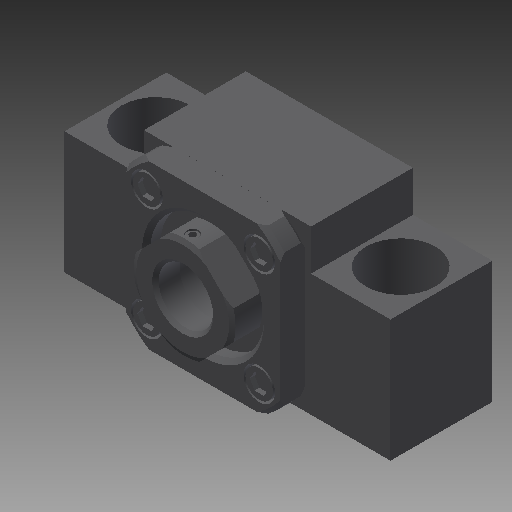
# Autodesk Inventor part: BK 15
Saved by Autodesk Inventor 2018 (Build 220112000, 112)
## iProperties
Category: PARTsolutions
Company: THK
Created: 2017-05-30
Part Number: BK 15
Catalog Web Link: www.cadenas.de
Description: Fixed Side type BK-
Vendor: THK
Document SubType Name: Modeling
Designer: psAdmin
Manufacturer: THK
Mass: 63.686 g
Surface Area: 225.318 cm^2
Volume: 63.686 cm^3
Density: 1 g/cm^3
Material: Generic
Appearance: PSOLRGB-192-192-192
PSOL_IDENT_0: {$CADENAS_DATA\23d-libs\thk\fed_screw\ball_screw\ball_screw_peripheral\suport_unit\fixed_side_type_b
PSOL_IDENT_1: k.prj},164 {VTYP=3D},{NB=BK 15},{LINA=BK 15},{NN=Fixed Side type BK},{DATE=16.05.2017 06:09:49},{GEO
PSOL_IDENT_2: MDATE=23.05.2016 07:00:00},{VERSION=},{LINEID=30},{LINESUBID=-1},{WBVAR=}  {NB=BK 15},{LINA=BK 15},{
PSOL_IDENT_3: KT=DUMMY},{IDNR=},{MN=BK 15},{SD=15.000},{L=27.000},{L1=6.000},{L2=32.000},{L3=6.000},{B=70.000},{H=
PSOL_IDENT_4: 48.000},{SB=35.000},{SH1=28.000},{B1=40.000},{H1=38.000},{E=18.000},{P=54.000},{C1=15.000},{C2=6.000
PSOL_IDENT_5: },{SD3=5.500},{SD1=6.600},{SD2=11.000},{SH=6.500},{NDM=3.000},{T=22.000},{DK=30.000},{L4=3.500},{SD4=
PSOL_IDENT_6: 19.500},{D=28.000},{DD=25.000},{P1=1.500},{PCD=39.000},{PCD1=49.500},{B2=38.000},{D1=7.800},{WF=4.00
PSOL_IDENT_7: 0},{WF1=1.500},{R3=25.000}
NN: Fixed side type BK
NB: BK 15
NBSYN: $MN.
LINA: BK 15
MN: BK 15
SUPPLIER: THK
ARTICLENO: BK 15
BOMINFO: BK 15
CREATOR: CADENAS GmbH
Title: BK 15
Author: Cadenas PARTsolutions
Autodesk Inventor part; units mm, degrees
sketch "Sketch_1" plane through (0, 0, 0) normal (0, 0, 1) x (1, 0, 0)
  line L0 (-40, -20) -> (40, -20)
  line L1 (40, -20) -> (40, 10)
  line L2 (40, 10) -> (20.5, 10)
  line L3 (20.5, 10) -> (20.5, 20)
  line L4 (20.5, 20) -> (-20.5, 20)
  line L5 (-20.5, 20) -> (-20.5, 10)
  line L6 (-20.5, 10) -> (-40, 10)
  line L7 (-40, 10) -> (-40, -20)
  line L8 (0, 20) -> (0, -20) construction
  line L9 (0, 20) -> (0, 0) construction
  dimension "d87" = 80
  dimension "d88" = 40
  dimension "d90" = 41
  dimension "d98" = 20
  dimension "d108" = 10
  constraints: 20 end point, 4 vertical, 2 horizontal, 2 midpoint, 1 collinear, 1 perpendicular, 1 other
  measures "d87" distance between parallel lines of L7 L1
  measures "d88" distance between parallel lines of L0 L4
  measures "d90" distance of L3.end L4.end
  measures "d98" distance from line of L9.end L4
  measures "d108" distance between parallel lines of L4 L2
extrude "Extrusion1" add sketch "Sketch_1" against normal blind 25
sketch "Sketch2" plane through (20.5, 10, 0) normal (0, 1, 0) x (1, 0, 0)
  line L0 (9.5, 12.5) -> (19.5, 12.5) construction
  line L1 (19.5, 0) -> (19.5, 25) projected
  dimension "d97" = 10
  constraints: 2 end point, 1 horizontal, 1 midpoint
  measures "d97" distance of L0.start L0.end
hole "Hole1" at (30, 10, -12.5) direction (0, -1, 0) diameter 11 end through all counterbore diameter 17 counterbore depth 15
sketch "Sketch_10" plane through (0, 0, 0) normal (0, 0, 1) x (1, 0, 0)
  line L0 (-19, 20) -> (-19, -20)
  line L1 (-19, -20) -> (19, -20)
  line L2 (19, -20) -> (19, 20)
  line L3 (19, 20) -> (-19, 20)
  constraints: 8 end point
extrude "Extrusion2" add sketch "Sketch_10" along normal blind 2.5
sketch "Sketch_13" plane through (0, 0, 0) normal (1, 0, 0) x (0, 1, 0)
  line L0 (0, 2.5) -> (0, 11)
  line L1 (0, 11) -> (12.5, 11)
  line L2 (12.5, 11) -> (12.5, 3.5)
  line L3 (12.5, 3.5) -> (10, 3.5)
  line L4 (10, 3.5) -> (10, 3)
  line L5 (10, 3) -> (9, 3)
  line L6 (9, 3) -> (9, 2.5)
  line L7 (9, 2.5) -> (0, 2.5)
  line L8 (0, 2.5) -> (0, 11)
  constraints: 18 end point
revolve "Revolution1" add sketch "Sketch_13" angle 360 about axis through (0, 0, 2.5) along (0, 0, -1)
sketch "Sketch_11" plane through (0, 0, 11) normal (0, 0, 1) x (1, 0, 0)
  line L0 (-22, 22) -> (-22, -22)
  line L1 (-22, -22) -> (22, -22)
  line L2 (22, -22) -> (22, 22)
  line L3 (22, 22) -> (-22, 22)
  line L4 (-15.5563, 0) -> (0, -15.5563)
  line L5 (0, -15.5563) -> (15.5563, 0)
  line L6 (15.5563, 0) -> (0, 15.5563)
  line L7 (0, 15.5563) -> (-15.5563, 0)
  constraints: 16 end point
extrude "Extrusion3" cut sketch "Sketch_11" against normal blind 8.5
sketch "Sketch_12" plane through (0, 0, 2.5) normal (0, 0, 1) x (1, 0, 0)
  line L0 (-19, 20) -> (-19, -20)
  line L1 (-19, -20) -> (19, -20)
  line L2 (19, -20) -> (19, 20)
  line L3 (19, 20) -> (-19, 20)
  circle A0 centre (0, 0) radius 14
  line L4 (-19, 20) -> (19, 20) projected
  line L5 (0, 20) -> (0, 20) construction
  line L6 (-20.5, 20) -> (20.5, 20) projected
  dimension "d91" = 28
  dimension "d92" = 38
  dimension "d93" = 38
  dimension "d94" = 40
  dimension "d95" = 40
  constraints: 10 end point, 2 midpoint, 1 centre point, 1 vertical
  measures "d91" diameter of A0
  measures "d92" distance of L2.end L0.start
  measures "d93" distance of L0.end L1.end
  measures "d94" distance of L0.start L0.end
  measures "d95" distance of L1.end L2.end
extrude "Extrusion4" add sketch "Sketch_12" along normal blind 3.5
sketch "Sketch_14" plane through (0, 0, 0) normal (1, 0, 0) x (0, 1, 0)
  line L0 (0, -50) -> (0, 50)
  line L1 (15, 6) -> (14, 6)
  line L2 (14, 6) -> (14, 5)
  line L3 (14, 5) -> (15, 6)
  constraints: 8 end point
revolve "Revolution2" cut sketch "Sketch_14" angle 360 about axis through (0, 0, -50) along (0, 0, -1)
sketch "Sketch11" plane through (0, 0, -25) normal (0, 0, -1) x (-1, 0, 0)
  point P0 (0, 0)
hole "Hole5" at (0, 0, -25) direction (0, 0, 1) diameter 15 depth 30 counterbore diameter 19.5 counterbore depth 6
sketch "Sketch_16" plane through (0, 0, 0) normal (1, 0, 0) x (0, 1, 0)
  line L0 (0, 2.5) -> (0, 11)
  line L1 (0, 11) -> (7.5, 11)
  line L2 (7.5, 11) -> (6.688, 10.188)
  line L3 (6.688, 10.188) -> (6.688, 3.312)
  line L4 (6.688, 3.312) -> (7.5, 2.5)
  line L5 (7.5, 2.5) -> (0, 2.5)
  line L6 (0, 2.5) -> (0, 11)
  constraints: 14 end point
revolve "Revolution3" cut sketch "Sketch_16" angle 360 about axis through (0, 0, 2.5) along (0, 0, -1)
thread "Thread1" size "M15x1.5" class "6H" standard "ISO Metric profile" full length
sketch "Sketch_17" plane through (0, 0, 0) normal (1, 0, 0) x (0, 1, 0)
  line L0 (0, -50) -> (0, 50)
  line L1 (14.05, 0) -> (14, 0)
  line L2 (14, 0) -> (14, -27)
  line L3 (14, -27) -> (14.05, -27)
  line L4 (14.05, -27) -> (14.05, 0)
  constraints: 10 end point
revolve "Revolution4" cut sketch "Sketch_17" angle 360 about axis through (0, 0, -50) along (0, 0, -1)
sketch "Sketch_18" plane through (0, 0, 0) normal (0.7071068, -0.7071068, 0) x (0, 0, -1)
  line L0 (-3, 19.5) -> (-6, 19.5)
  line L1 (-6, 19.5) -> (-6, 23.4)
  line L2 (-6, 23.4) -> (-3, 23.4)
  line L3 (-3, 23.4) -> (-3, 19.5)
  line L4 (-3, 19.5) -> (-6, 19.5)
  constraints: 10 end point
revolve "Revolution5" cut sketch "Sketch_18" angle 360 about axis through (13.7886, 13.7886, 3) along (0, 0, -1)
pattern_linear "Rectangular Pattern1" count 2 spacing 27.5772 along (-1, 0, 0) count 2 spacing 27.5772 along (0, -1, 0) of "Revolution5"
sketch "Sketch_20" plane through (0, 0, 0) normal (0.7071068, -0.7071068, 0) x (0, 0, -1)
  line L0 (-3, 19.5) -> (-6, 19.5)
  line L1 (-6, 19.5) -> (-6, 22.9)
  line L2 (-6, 22.9) -> (-3, 22.9)
  line L3 (-3, 22.9) -> (-3, 19.5)
  line L4 (-3, 19.5) -> (-6, 19.5)
  constraints: 10 end point
revolve "Revolution6" add sketch "Sketch_20" angle 360 about axis through (13.7886, 13.7886, 3) along (0, 0, -1)
pattern_linear "Rectangular Pattern2" count 2 spacing 27.5772 along (-1, 0, 0) count 2 spacing 27.5772 along (0, -1, 0) of "Revolution6"
sketch "Sketch_22" plane through (0, 0, 6) normal (0, 0, 1) x (0.7071068, 0.7071068, 0)
  line L0 (17.2693, -0.5977) -> (18.9023, -2.2307)
  line L1 (18.9023, -2.2307) -> (21.133, -1.633)
  line L2 (21.133, -1.633) -> (21.7307, 0.5977)
  line L3 (21.7307, 0.5977) -> (20.0977, 2.2307)
  line L4 (20.0977, 2.2307) -> (17.867, 1.633)
  line L5 (17.867, 1.633) -> (17.2693, -0.5977)
  constraints: 12 end point
extrude "Extrusion5" cut sketch "Sketch_22" against normal blind 1.2
pattern_linear "Rectangular Pattern3" count 2 spacing 27.5772 along (-1, 0, 0) count 2 spacing 27.5772 along (0, -1, 0) of "Extrusion5"
sketch "Sketch_24" plane through (0, 0, 0) normal (1, 0, 0) x (0, 1, 0)
  line L0 (12.5, 8.5) -> (7.5, 8.5)
  line L1 (7.5, 8.5) -> (7.5, 10)
  line L2 (7.5, 10) -> (12.5, 10)
  line L3 (12.5, 10) -> (12.5, 8.5)
  line L4 (12.5, 8.5) -> (7.5, 8.5)
  constraints: 10 end point
revolve "Revolution7" cut sketch "Sketch_24" angle 360 about axis through (0, 12.5, 8.5) along (0, 1, 0)
sketch "Sketch_25" plane through (0, 0, 0) normal (1, 0, 0) x (0, 1, 0)
  line L0 (12.3, 8.5) -> (8.8, 8.5)
  line L1 (8.8, 8.5) -> (8.8, 10)
  line L2 (8.8, 10) -> (12, 10)
  arc A0 (12.3, 9.7) -> (12, 10) centre (12, 9.7) ccw
  line L3 (12.3, 9.7) -> (12.3, 8.5)
  line L4 (12.3, 8.5) -> (8.8, 8.5)
  constraints: 10 end point, 2 point on circle, 1 centre point
revolve "Revolution8" add sketch "Sketch_25" angle 360 about axis through (0, 12.3, 8.5) along (0, 1, 0)
sketch "Sketch_26" plane through (0, 12.3, 0) normal (0, 1, 0) x (1, 0, 0)
  line L0 (-0.75, -8.933) -> (0, -9.366)
  line L1 (0, -9.366) -> (0.75, -8.933)
  line L2 (0.75, -8.933) -> (0.75, -8.067)
  line L3 (0.75, -8.067) -> (0, -7.634)
  line L4 (0, -7.634) -> (-0.75, -8.067)
  line L5 (-0.75, -8.067) -> (-0.75, -8.933)
  constraints: 12 end point
extrude "Extrusion6" cut sketch "Sketch_26" against normal blind 1.2
sketch "Sketch_28" plane through (0, 0, 0) normal (1, 0, 0) x (0, 1, 0)
  line L0 (0, -50) -> (0, 50)
  line L1 (11.4, 11) -> (12.5, 10.5)
  line L2 (12.5, 10.5) -> (12.5, 11)
  line L3 (12.5, 11) -> (11.4, 11)
  constraints: 8 end point
revolve "Revolution9" cut sketch "Sketch_28" angle 360 about axis through (0, 0, -50) along (0, 0, -1)
sketch "Sketch_29" plane through (0, 0, 0) normal (1, 0, 0) x (0, 1, 0)
  line L0 (0, -50) -> (0, 50)
  line L1 (12.5, 4) -> (11.4, 3.5)
  line L2 (11.4, 3.5) -> (12.5, 3.5)
  line L3 (12.5, 3.5) -> (12.5, 4)
  constraints: 8 end point
revolve "Revolution10" cut sketch "Sketch_29" angle 360 about axis through (0, 0, -50) along (0, 0, -1)
sketch "Sketch_33" plane through (0, 0, 0) normal (0.7071068, 0.7071068, 0) x (0, 0, -1)
  line L0 (50, 0) -> (-50, 0)
  line L1 (-6, 24.75) -> (-4.5, 27.25)
  line L2 (-4.5, 27.25) -> (-6, 27.25)
  line L3 (-6, 27.25) -> (-6, 24.75)
  constraints: 8 end point
extrude "Extrusion7" cut sketch "Sketch_33" along normal mid plane 16
sketch "Sketch_27" plane through (0, 0, 0) normal (0, 0, 1) x (1, 0, 0)
  line L0 (-40, 40) -> (-40, -40)
  line L1 (-40, -40) -> (40, -40)
  line L2 (40, -40) -> (40, 40)
  line L3 (40, 40) -> (-40, 40)
  circle A0 centre (0, 0) radius 25
  constraints: 8 end point, 1 centre point
extrude "Extrusion8" cut sketch "Sketch_27" along normal blind 6
sketch "Sketch_30" plane through (0, 0, 0) normal (1, 0, 0) x (0, 1, 0)
  line L0 (0, -50) -> (0, 50)
  line L1 (24, 6) -> (25, 5)
  line L2 (25, 5) -> (25, 6)
  line L3 (25, 6) -> (24, 6)
  constraints: 8 end point
revolve "Revolution11" cut sketch "Sketch_30" angle 360 about axis through (0, 0, -50) along (0, 0, -1)
sketch "Sketch_31" plane through (0, 0, 0) normal (1, 0, 0) x (0, 1, 0)
  line L0 (0, -50) -> (0, 50)
  line L1 (25, 1) -> (24, 0)
  line L2 (24, 0) -> (25, 0)
  line L3 (25, 0) -> (25, 1)
  constraints: 8 end point
revolve "Revolution12" cut sketch "Sketch_31" angle 360 about axis through (0, 0, -50) along (0, 0, -1)
sketch "Sketch_32" plane through (0, 0, 0) normal (0, 0, 1) x (1, 0, 0)
  line L0 (-40, -40) -> (40, -40)
  line L1 (40, -40) -> (40, 40)
  line L2 (40, 40) -> (-40, 40)
  line L3 (-40, 40) -> (-40, -40)
  line L4 (-18.98, 19.98) -> (-18.98, -19.98)
  line L5 (-18.98, -19.98) -> (18.98, -19.98)
  line L6 (18.98, -19.98) -> (18.98, 19.98)
  line L7 (18.98, 19.98) -> (-18.98, 19.98)
  constraints: 16 end point
extrude "Extrusion9" cut sketch "Sketch_32" along normal blind 0.01
ref_plane "unit_XY" through (0, 0, 0) normal (0, 0, -1) x (1, 0, 0)
ref_plane "unit_YZ" through (0, 0, 0) normal (1, 0, 0) x (0, -1, 0)
ref_plane "unit_ZX" through (0, 0, 0) normal (0, -1, 0) x (0, 0, -1)
ref_plane "unit_collar_XY" through (0, 0, -21) normal (0, 0, 1) x (1, 0, 0)
ref_plane "unit_collar_YZ" through (0, 0, -21) normal (1, 0, 0) x (0, 1, 0)
ref_plane "unit_collar_ZX" through (0, 0, -21) normal (0, 1, 0) x (0, 0, 1)
sketch "Sketch27" plane through (-39.75, 10, 0) normal (0, 1, 0) x (1, 0, 0)
  line L0 (19.7564, -0.3205) -> (19.7564, 25.3205)
  line L1 (9.75, 12.5) -> (-0.25, 12.5) construction
  line L2 (-0.25, 0) -> (-0.25, 25) projected
  dimension "d107" = 10
  constraints: 4 end point, 1 midpoint
  measures "d107" distance of L1.start L1.end
hole "Hole6" at (-30, 10, -12.5) direction (0, -1, 0) diameter 11 end through all counterbore diameter 17 counterbore depth 15
body "Solid1"
